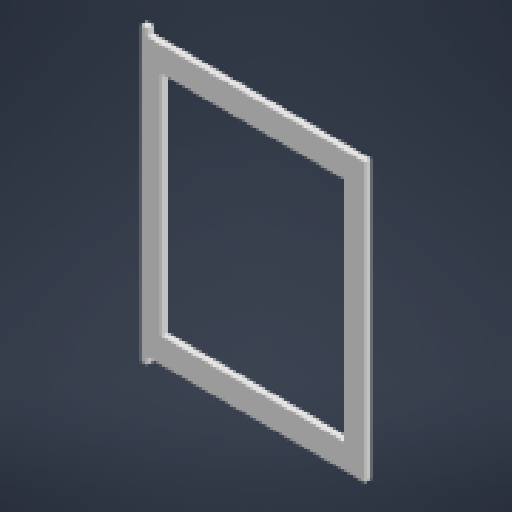
# Autodesk Inventor part: Pieza10
Saved by Autodesk Inventor 2026.1 (Build 301233020, 233B)
## iProperties
Created: 2026-05-06
Part Number: Pieza10
Material: Genérico
Document SubType Name: Modeling
Designer: OlmesTech
Density: 1 g/cm^3
Appearance: Valor por defecto
Author: OlmesTech
Autodesk Inventor part; units mm, degrees
ref_plane "YZ Plane" through (0, 0, 0) normal (1, 0, 0) x (0, 1, 0)
ref_plane "XZ Plane" through (0, 0, 0) normal (0, 1, 0) x (-1, 0, 0)
ref_plane "XY Plane" through (0, 0, 0) normal (0, 0, 1) x (1, 0, 0)
sketch "Boceto1" plane through (0, 0, 0) normal (0, 0, 1) x (1, 0, 0)
  line L0 (0, 0) -> (0, -127) projected
  line L1 (0, -130) -> (0, -127) projected
  line L2 (-101.4948, -130) -> (-101.4948, -133)
  line L3 (-101.4948, 3) -> (-101.4948, 0)
  line L4 (-104.4221, 0) -> (-104.4221, -130)
  line L5 (-104.4221, -133) -> (-101.4948, -133)
  line L6 (-104.4221, 3) -> (-101.4948, 3)
  line L7 (-9.639, -118) -> (-94.7832, -118)
  line L8 (-94.7832, -118) -> (-94.7832, -12)
  line L9 (-94.7832, -12) -> (-9.639, -12)
  line L10 (-9.639, -12) -> (-9.639, -118)
  line L11 (-9.639, -118) -> (-94.7832, -12) construction
  line L12 (-94.7832, -118) -> (-9.639, -12) construction
  line L13 (-104.4221, -133) -> (-104.4221, -130)
  line L14 (-104.4221, 0) -> (-104.4221, 3)
  line L15 (-101.4948, -130) -> (-101.4948, -129.7)
  line L16 (-101.4948, -129.7) -> (0, -129.7)
  line L17 (-101.4948, 0) -> (-101.4948, -0.3)
  line L18 (-101.4948, -0.3) -> (0, -0.3)
  point P0 (-2.2595, 0)
  dimension "d3" = 9.639
  dimension "d4" = 0.3
  dimension "d5" = 0.3
  constraints: 34 end point, 5 point on line, 4 perpendicular, 4 vertical, 3 parallel, 1 collinear, 1 horizontal, 4 other
  measures "d3" distance between parallel lines of L4 L8
  measures "d4" distance of L15.start L15.end
  measures "d5" distance of L17.start L17.end
extrude "Extrusión1" add sketch "Boceto1" along normal blind 3
